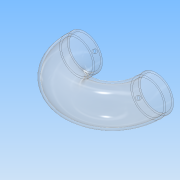
# Autodesk Inventor part: Pancake_Flexi Pipe Flipped
Saved by Autodesk Inventor 2018.1 (Build 221171000, 171)
## iProperties
Created: 2019-02-26
Part Number: Pancake_Flexi Pipe Flipped
Material: PMMA Plastic
Document SubType Name: Modeling
Designer: James
Density: 1.188 g/cm^3
Appearance: Polycarbonate - Clear
Mass: 64.5196 g
Surface Area: 441.857 cm^2
Volume: 54.3094 cm^3
Author: James
Autodesk Inventor part; units mm, degrees
note: some values were not read from the file. Chosen so that the rebuilt part matches the saved one: direction of "Hole1".
ref_plane "XZ Plane" through (0, 0, 0) normal (0, 1, 0) x (-1, 0, 0)
ref_plane "XY Plane" through (0, 0, 0) normal (0, 0, 1) x (1, 0, 0)
sketch "Sketch1" plane through (0, 0, 0) normal (0, 1, 0) x (-1, 0, 0)
  circle A0 centre (0, 0) radius 20
  circle A1 centre (0, 0) radius 22.5
  dimension "d0" = 40
  dimension "d1" = 45
  constraints: 2 centre point, 2 coincident
  measures "d0" diameter of A0
  measures "d1" diameter of A1
sketch "Sketch2" plane through (0, 0, 0) normal (0, 0, 1) x (1, 0, 0)
  arc A0 (-91, 0) -> (0, 0) centre (-45.5, 0) ccw
  dimension "d34" = 91
  constraints: 2 horizontal alignment, 2 point on circle, 1 centre point
  measures "d34" distance of A0.end A0.start
sweep "Sweep2" add profiles "Sketch1" path "Sketch2"
sketch "Sketch3" plane through (-91, 0, 0) normal (0, 1, 0) x (1, 0, 0)
  circle A0 centre (0, 0) radius 20 projected
  circle A1 centre (0, 0) radius 22.5 projected
  circle A2 centre (91, 0) radius 20 projected
  circle A3 centre (91, 0) radius 22.5 projected
extrude "Extrusion1" add sketch "Sketch3" along normal blind 10
ref_plane "Work Plane1" through (0, 0, 0) normal (0.8290376, 0, 0.5591929) x (0, 1, 0)
sketch "Sketch4" plane through (0, 0, 0) normal (0.8290376, 0, 0.5591929) x (0, 1, 0)
  line L0 (10, -22.5) -> (10, 22.5) projected
  line L1 (0, 22.5) -> (0, -22.5) projected
  point P0 (0, 0)
  point P1 (5, 0)
  dimension "d14" = 5
  dimension "d15" = 22.5
  dimension "d16" = 22.5
  measures "d14" distance from line of L0 point (5, 0)
  measures "d15" vertical distance of L0.start point (5, 0)
  measures "d16" vertical distance of L0.end point (5, 0)
hole "Hole1" at (0, 5, 0) direction (-0.8290376, 0, -0.5591929) diameter 4.5 end up to surface
sketch "Sketch5" plane through (-91, 10, 0) normal (0, 1, 0) x (1, 0, 0)
  point P0 (91, 0)
  point P1 (0, 0)
  point P2 (0, 0)
  constraints: 1 coincident
ref_plane "Work Plane2" through (-91, 10, 0) normal (0.8290376, 0, 0.5591929) x (0, 1, 0)
sketch "Sketch6" plane through (-91, 10, 0) normal (0.8290376, 0, 0.5591929) x (0, 1, 0)
  line L0 (0, -22.5) -> (0, 22.5) projected
  line L1 (-10, -22.5) -> (-10, 22.5) projected
  line L2 (-10, -22.5) -> (0, -22.5) projected
  line L3 (-10, 22.5) -> (0, 22.5) projected
  point P0 (-10, -50.8866)
  point P1 (-5, 0)
  dimension "d24" = 5
  dimension "d25" = 22.5
  dimension "d26" = 22.5
  measures "d24" distance from line of L0 point (-5, 0)
  measures "d25" distance from line of point (-5, 0) L2
  measures "d26" distance from line of point (-5, 0) L3
hole "Hole2" at (-91, 5, 0) direction (0.8290376, 0, 0.5591929) diameter 4.5 end up to surface
equation "\"d15\" = d16"
equation "\"d25\" = d26"
body "Solid2"
